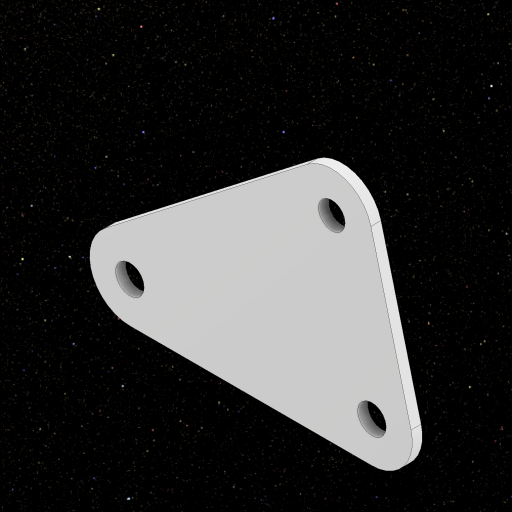
# Autodesk Inventor part: odom_pod
Saved by Autodesk Inventor 2024 (Build 280153000, 153)
## iProperties
Created: 2024-02-24
Part Number: odom_pod
Material: Acetal Resin, White
Document SubType Name: Modeling
Designer: Averey Ku
Density: 1.425 g/cm^3
Appearance: Smooth - White
Author: Averey Ku
Autodesk Inventor part; units mm, degrees
ref_plane "YZ Plane" through (0, 0, 0) normal (1, 0, 0) x (0, 1, 0)
ref_plane "XZ Plane" through (0, 0, 0) normal (0, 1, 0) x (-1, 0, 0)
ref_plane "XY Plane" through (0, 0, 0) normal (0, 0, 1) x (1, 0, 0)
sketch "Sketch1" plane through (0, 0, 0) normal (0, 0, 1) x (1, 0, 0)
  circle A0 centre (0, 0) radius 2.2479
  circle A1 centre (38.1, 0) radius 2.2479
  circle A2 centre (31.7833, 24.602) radius 2.0955
  arc A3 (-3.8869, 5.0214) -> (0, -6.35) centre (0, 0) ccw
  arc A4 (37.9338, 26.1812) -> (27.8964, 29.6234) centre (31.7833, 24.602) ccw
  arc A5 (38.1, -6.35) -> (44.2505, 1.5792) centre (38.1, 0) ccw
  line L0 (-3.8869, 5.0214) -> (27.8964, 29.6234)
  line L1 (37.9338, 26.1812) -> (44.2505, 1.5792)
  line L2 (0, -6.35) -> (38.1, -6.35)
  line L3 (38.1, 0) -> (63.5, 0) construction
  dimension "d0" = 4.4958
  dimension "d5" = 12.7
  dimension "d6" = 12.7
  dimension "d7" = 12.7
  constraints: 8 end point, 6 centre point, 6 point on circle, 5 tangent, 4 coincident, 1 horizontal, 1 other
  measures "d0" diameter of A0
  measures "d5" diameter of A3
  measures "d6" diameter of A4
  measures "d7" diameter of A5
extrude "Extrusion1" add sketch "Sketch1" along normal blind 1.5875
body "Solid1"
